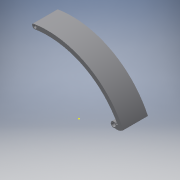
# Autodesk Inventor part: battery gate
Saved by Autodesk Inventor 2016 (Build 200138000, 138)
## iProperties
Created: 2015-08-20
Part Number: battery gate
Material: Generic
Document SubType Name: Modeling
Designer: TFHulbert
Density: 1 g/cm^3
Appearance: Default
Author: TFHulbert
Autodesk Inventor part; units mm, degrees
ref_plane "YZ Plane" through (0, 0, 0) normal (1, 0, 0) x (0, 1, 0)
ref_plane "XZ Plane" through (0, 0, 0) normal (0, 1, 0) x (-1, 0, 0)
ref_plane "XY Plane" through (0, 0, 0) normal (0, 0, 1) x (1, 0, 0)
sketch "Sketch1" plane through (0, 0, 0) normal (0, 1, 0) x (-1, 0, 0)
  arc A0 (31.5311, 101.5419) -> (30.2114, 104.4989) centre (29.799, 102.5419) ccw
  arc A1 (-91.2437, 34.3767) -> (-89.3427, 31.7554) centre (-89.3427, 33.7554) ccw
  line L0 (31.5311, 101.5419) -> (23.8911, 88.309)
  arc A2 (23.8911, 88.309) -> (24.6231, 85.577) centre (25.6231, 87.309) ccw
  line L1 (-89.3427, 31.7554) -> (-74.0627, 31.7554)
  arc A3 (-72.0627, 29.7554) -> (-74.0627, 31.7554) centre (-74.0627, 29.7554) ccw
  arc A4 (30.2114, 104.4989) -> (-91.2437, 34.3767) centre (8.5603, 1.7554) ccw
  circle A5 centre (-72.0627, 44.7554) radius 2.5
  arc A6 (28.2386, 101.8391) -> (-83.9329, 44.7554) centre (8.5603, 1.7554) ccw
  line L2 (28.2386, 101.8391) -> (25.4884, 97.0757)
  arc A7 (-83.9329, 44.7554) -> (-73.5865, 41.7466) centre (-76.1912, 52.0832) ccw
  arc A8 (25.4884, 97.0757) -> (-77.185, 46.7026) centre (8.5603, 1.7554) ccw
  arc A9 (-77.185, 46.7026) -> (-75.0545, 46.3123) centre (-75.4078, 50.3936) ccw
  line L3 (29.799, 102.5419) -> (29.799, 100.0419)
  line L4 (29.799, 100.0419) -> (23.799, 100.0419)
  circle A10 centre (23.799, 100.0419) radius 2
  arc A11 (-73.5865, 41.7466) -> (-75.0545, 46.3123) centre (-72.0627, 44.7554) ccw
  dimension "d6" = 5
  dimension "d10" = 3
  dimension "d11" = 2.5
  dimension "d12" = 6
  dimension "d13" = 4
  constraints: 20 point on circle, 12 centre point, 10 end point, 1 coincident, 1 perpendicular, 1 vertical
  measures "d6" diameter of A5
  measures "d10" radial gap between concentric circles of A4 A6
  measures "d11" distance of L3.start L3.end
  measures "d12" distance of L3.end L4.end
  measures "d13" diameter of A10
extrude "Extrusion3" add sketch "Sketch1" along normal blind 30
fillet "Fillet1" radius 2 2 edges at (-28.2386, 15, 101.8391) (-25.4884, 15, 97.0757)
sketch "Sketch3" plane through (0, 30, 0) normal (0, 1, 0) x (1, 0, 0)
  point P0 (0, 0)
sketch "Sketch4" plane through (0, 30, 0) normal (0, 1, 0) x (1, 0, 0)
  point P0 (0, 0)
ref_plane "Work Plane1" through (0, 10, 0) normal (0, -1, 0) x (1, 0, 0)
sketch "Sketch6" plane through (0, 10, 0) normal (0, -1, 0) x (1, 0, 0)
  circle A0 centre (-23.799, 100.0419) radius 2 projected
  circle A1 centre (-23.799, 100.0419) radius 1.5
  point P0 (0, 0)
  dimension "d19" = 3
  constraints: 1 centre point, 1 coincident
  measures "d19" diameter of A1
extrude "Extrusion4" add sketch "Sketch6" along normal blind 2
body "Solid2"
